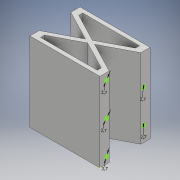
# Autodesk Inventor part: legspacer_paula_v2
Saved by Autodesk Inventor 2018 (Build 220112000, 112)
## iProperties
Created: 2020-03-09
Part Number: legspacer_paula_v2
Material: Generic
Document SubType Name: Modeling
Designer: bitbots
Density: 1 g/cm^3
Appearance: Default
Author: bitbots
Autodesk Inventor part; units mm, degrees
ref_plane "YZ Plane" through (0, 0, 0) normal (1, 0, 0) x (0, 1, 0)
ref_plane "XZ Plane" through (0, 0, 0) normal (0, 1, 0) x (-1, 0, 0)
ref_plane "XY Plane" through (0, 0, 0) normal (0, 0, 1) x (1, 0, 0)
sketch "Sketch1" plane through (0, 0, 0) normal (0, 0, 1) x (1, 0, 0)
  line L0 (0, 0) -> (53, 0)
  line L1 (53, 0) -> (53, 38) construction
  line L2 (53, 38) -> (0, 38)
  line L3 (0, 38) -> (0, 0) construction
  line L4 (5, 35) -> (48, 35)
  line L5 (48, 3) -> (5, 3)
  line L6 (53, 7) -> (0, 7) construction
  line L7 (0, 31) -> (53, 31) construction
  line L8 (5, 38) -> (5, 0) construction
  line L9 (48, 38) -> (48, 0) construction
  line L10 (0, 31) -> (53, 31) construction
  line L11 (0, 31) -> (53, 31) construction
  line L12 (0, 31) -> (54.1143, 31) construction
  line L13 (53, 7) -> (107.1143, 7) construction
  line L14 (0, 31) -> (53.8717, 31) construction
  line L15 (53, 7) -> (106.8717, 7) construction
  line L16 (0, 31) -> (48, 6.0128) construction
  line L17 (0, 31) -> (54.1143, 31) construction
  line L18 (53, 7) -> (5, 31.9872) construction
  line L19 (53, 7) -> (107.1143, 7) construction
  line L20 (53, 38) -> (53, 31)
  line L21 (0, 38) -> (0, 31)
  line L22 (0, 7) -> (0, 0)
  line L23 (53, 7) -> (53, 0)
  line L24 (0, 7) -> (48, 31.9872) construction
  line L25 (0, 7) -> (54.1143, 7) construction
  line L26 (53, 31) -> (5, 6.0128) construction
  line L27 (53, 31) -> (107.1143, 31) construction
  line L28 (5, 35) -> (5, 31.9872)
  line L29 (48, 35) -> (48, 31.9872)
  line L30 (5, 6.0128) -> (5, 3)
  line L31 (48, 6.0128) -> (48, 3)
  line L32 (5, 31.9872) -> (26.5, 20.795)
  line L33 (48, 6.0128) -> (26.5, 17.205)
  line L34 (23.0518, 19) -> (0, 31)
  line L35 (0, 7) -> (23.0518, 19)
  line L36 (26.5, 20.795) -> (48, 31.9872)
  line L37 (26.5, 17.205) -> (5, 6.0128)
  line L38 (29.9482, 19) -> (53, 31)
  line L39 (53, 7) -> (29.9482, 19)
  dimension "d12" = 53
  dimension "d13" = 38
  dimension "d14" = 3
  dimension "d15" = 3
  dimension "d16" = 4
  dimension "d17" = 4
  dimension "d18" = 5
  dimension "d19" = 5
  dimension "d27" = 27.5
  dimension "d28" = 152.5
  dimension "d29" = 27.5
  dimension "d30" = 152.5
  constraints: 80 end point, 20 point on line, 12 collinear, 11 horizontal, 4 equal length, 4 parallel, 2 coincident, 2 perpendicular
  measures "d12" distance of L2.end L1.end
  measures "d13" distance of L1.end L0.end
  measures "d14" distance between parallel lines of L2 L4
  measures "d15" distance between parallel lines of L0 L5
  measures "d16" distance between parallel lines of L5 L6
  measures "d17" distance between parallel lines of L4 L7
  measures "d18" distance between parallel lines of L3 L8
  measures "d19" distance between parallel lines of L1 L9
  measures "d27" angle of L16 L17
  measures "d28" angle of L19 L18
  measures "d29" angle of L25 L24
  measures "d30" angle of L26 L27
extrude "Extrusion1" add sketch "Sketch1" along normal blind 60
sketch "Sketch2" plane through (53, 0, 0) normal (1, 0, 0) x (0, 0, -1)
  circle A0 centre (-55, 5) radius 1.35
  circle A1 centre (-30, 5) radius 1.35
  circle A2 centre (-5, 5) radius 1.35
  circle A3 centre (-36.465, 33) radius 1.35
  circle A4 centre (-11.465, 33) radius 1.35
  point P0 (0, 0)
  dimension "d33" = 2.7
  dimension "d34" = 2.7
  dimension "d35" = 2.7
  dimension "d36" = 2.7
  dimension "d37" = 2.7
  constraints: 5 centre point, 5 coincident
  measures "d33" diameter of A0
  measures "d34" diameter of A1
  measures "d35" diameter of A2
  measures "d36" diameter of A3
  measures "d37" diameter of A4
body "Solid1"
